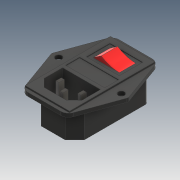
# Autodesk Inventor part: power-port
Saved by Autodesk Inventor 2017 (Build 210142000, 142)
## iProperties
Created: 2018-07-14
Part Number: power-port
Material: UHMW, Black
Document SubType Name: Modeling
Designer: Luiz Gustavo
Density: 0.94 g/cm^3
Appearance: Smooth - Black
Author: Luiz Gustavo
Autodesk Inventor part; units mm, degrees
ref_plane "YZ Plane" through (0, 0, 0) normal (1, 0, 0) x (0, 1, 0)
ref_plane "XZ Plane" through (0, 0, 0) normal (0, 1, 0) x (-1, 0, 0)
ref_plane "XY Plane" through (0, 0, 0) normal (0, 0, 1) x (1, 0, 0)
sketch "Sketch3" plane through (0, 0, 0) normal (0, 0, 1) x (1, 0, 0)
  line L0 (-13.75, 23.5) -> (13.75, 23.5)
  line L1 (13.75, 23.5) -> (13.75, -23.5)
  line L2 (13.75, -23.5) -> (-13.75, -23.5)
  line L3 (-13.75, -23.5) -> (-13.75, 23.5)
  line L4 (-13.75, 23.5) -> (13.75, -23.5) construction
  line L5 (13.75, 23.5) -> (-13.75, -23.5) construction
  point P0 (0, 0)
  dimension "d17" = 27.5
  dimension "d18" = 47
  constraints: 12 end point, 2 midpoint, 2 parallel, 1 horizontal, 1 perpendicular
  measures "d17" distance of L1.end L2.end
  measures "d18" distance between parallel lines of L2 L0
extrude "Extrusion1" add sketch "Sketch3" against normal blind 20
sketch "Sketch2" plane through (0, 0, 0) normal (0, 0, 1) x (1, 0, 0)
  line L0 (-24.5, 0) -> (24.5, 0) construction
  line L1 (0, 29.1) -> (0, -29.1) construction
  line L2 (-14, 29.1) -> (14, 29.1)
  line L3 (-14, 29.1) -> (-24.5, 0)
  line L4 (14, 29.1) -> (24.5, 0)
  line L5 (-14, -29.1) -> (14, -29.1)
  line L6 (-24.5, 0) -> (-14, -29.1)
  line L7 (24.5, 0) -> (14, -29.1)
  circle A0 centre (20, 0) radius 2
  circle A1 centre (-20, 0) radius 2
  point P0 (0, 0)
  point P1 (0, 0)
  dimension "d12" = 49
  dimension "d13" = 58.2
  dimension "d14" = 28
  dimension "d15" = 4
  dimension "d16" = 40
  constraints: 16 end point, 4 midpoint, 3 horizontal, 2 centre point, 2 point on line, 1 coincident, 1 equal radius, 1 parallel, 1 vertical, 1 other
  measures "d12" distance of L0.start L0.end
  measures "d13" distance of L1.start L1.end
  measures "d14" distance of L2.start L2.end
  measures "d15" diameter of A0
  measures "d16" distance of A1.centre A0.centre
extrude "Extrusion2" add sketch "Sketch2" against normal blind 2.3
sketch "Sketch1" plane through (0, 0, 0) normal (0, 0, 1) x (1, 0, 0)
  line L0 (-14.15, 27.2) -> (14.15, 27.2)
  line L1 (14.15, 27.2) -> (14.15, -27.2)
  line L2 (14.15, -27.2) -> (-14.15, -27.2)
  line L3 (-14.15, -27.2) -> (-14.15, 27.2)
  line L4 (-14.15, 27.2) -> (14.15, -27.2) construction
  line L5 (14.15, 27.2) -> (-14.15, -27.2) construction
  line L6 (-10.5, 23.2) -> (10.5, 23.2)
  line L7 (10.5, 23.2) -> (10.5, 8.2)
  line L8 (10.5, 8.2) -> (-10.5, 8.2)
  line L9 (-10.5, 8.2) -> (-10.5, 23.2)
  line L10 (-10.5, 23.2) -> (10.5, 8.2) construction
  line L11 (10.5, 23.2) -> (-10.5, 8.2) construction
  line L12 (0, 15.7) -> (0, 0) construction
  line L13 (-12.1, -5.4) -> (12.1, -5.4)
  line L14 (12.1, -5.4) -> (12.1, -22.2)
  line L15 (12.1, -22.2) -> (-12.1, -22.2)
  line L16 (-12.1, -22.2) -> (-12.1, -5.4)
  line L17 (-12.1, -5.4) -> (12.1, -22.2) construction
  line L18 (12.1, -5.4) -> (-12.1, -22.2) construction
  line L19 (0, 0) -> (0, -13.8) construction
  line L20 (-8.3, 20.95) -> (8.3, 20.95)
  line L21 (8.3, 20.95) -> (8.3, 10.45)
  line L22 (8.3, 10.45) -> (-8.3, 10.45)
  line L23 (-8.3, 10.45) -> (-8.3, 20.95)
  line L24 (-8.3, 20.95) -> (8.3, 10.45) construction
  line L25 (8.3, 20.95) -> (-8.3, 10.45) construction
  line L26 (-12.5, 5.8689) -> (12.5, 5.8689)
  line L27 (12.5, 5.8689) -> (12.5, -3.1311)
  line L28 (12.5, -3.1311) -> (-12.5, -3.1311)
  line L29 (-12.5, -3.1311) -> (-12.5, 5.8689)
  line L30 (-12.5, 5.8689) -> (12.5, -3.1311) construction
  line L31 (12.5, 5.8689) -> (-12.5, -3.1311) construction
  point P0 (0, 1.3689)
  dimension "d0" = 28.3
  dimension "d1" = 54.4
  dimension "d2" = 21
  dimension "d3" = 15
  dimension "d4" = 4
  dimension "d5" = 24.2
  dimension "d6" = 16.8
  dimension "d7" = 5
  dimension "d8" = 16.6
  dimension "d9" = 10.5
  dimension "d10" = 25
  dimension "d11" = 9
  constraints: 64 end point, 10 midpoint, 10 parallel, 5 horizontal, 5 perpendicular, 2 vertical, 1 point on line
  measures "d0" distance of L1.end L2.end
  measures "d1" distance of L0.end L1.end
  measures "d2" distance of L7.end L8.end
  measures "d3" distance of L6.end L7.end
  measures "d4" distance between parallel lines of L6 L0
  measures "d5" distance of L14.end L15.end
  measures "d6" distance of L13.end L14.end
  measures "d7" distance between parallel lines of L2 L15
  measures "d8" distance of L21.end L22.end
  measures "d9" distance of L20.end L21.end
  measures "d10" distance of L27.end L28.end
  measures "d11" distance of L26.end L27.end
extrude "Extrusion3" add sketch "Sketch1" along normal blind 1 contours L0 L1 L2 L3
extrude "Extrusion4" add sketch "Sketch1" along normal blind 0.5 contours L6 L7 L8 L9 | L26 L27 L28 L29
extrude "Extrusion5" add sketch "Sketch1" along normal blind 4 contours L20 L21 L22 L23
sketch "Sketch4" plane through (-8.3, 20.95, 0.5) normal (0, 1, 0) x (1, 0, 0)
  line L0 (0, -3.5) -> (16.6, -3.5) projected
  line L1 (0, 0) -> (0, -3.5) projected
  line L2 (16.6, 0) -> (16.6, -3.5) projected
  line L3 (0, 0) -> (5, -3.5)
  arc A0 (16.6, 0) -> (5, -3.5) centre (16.6082, -21) ccw
  point P0 (8.3, 0.5)
  dimension "d29" = 5
  dimension "d30" = 21
  constraints: 2 end point, 2 point on circle, 1 centre point, 1 point on line
  measures "d29" distance of L3.end L0.start
  measures "d30" radius of A0
extrude "Extrusion6" cut sketch "Sketch4" against normal up to surface (10.5 mm away)
extrude "Extrusion7" cut sketch "Sketch1" against normal blind 19 contours L13 L14 L15 L16
sketch "Sketch5" plane through (0, 0, 0) normal (0, 0, 1) x (1, 0, 0)
  line L0 (-1, -14.8319) -> (1, -14.8319)
  line L1 (1, -14.8319) -> (1, -18.3319)
  line L2 (1, -18.3319) -> (-1, -18.3319)
  line L3 (-1, -18.3319) -> (-1, -14.8319)
  line L4 (-8, -10.3319) -> (-6, -10.3319)
  line L5 (-6, -10.3319) -> (-6, -13.8319)
  line L6 (-6, -13.8319) -> (-8, -13.8319)
  line L7 (-8, -13.8319) -> (-8, -10.3319)
  line L8 (6, -10.3319) -> (8, -10.3319)
  line L9 (8, -10.3319) -> (8, -13.8319)
  line L10 (8, -13.8319) -> (6, -13.8319)
  line L11 (6, -13.8319) -> (6, -10.3319)
  line L12 (-8, -12.0819) -> (8, -12.0819) construction
  line L13 (0, -14.8319) -> (0, -12.0819) construction
  point P0 (0, 0)
  dimension "d35" = 2
  dimension "d36" = 3.5
  dimension "d42" = 16
  dimension "d43" = 8
  constraints: 28 end point, 10 parallel, 4 horizontal, 4 midpoint, 3 perpendicular, 1 vertical
  measures "d35" distance of L1.end L2.end
  measures "d36" distance of L0.end L1.end
  measures "d42" distance of L12.start L12.end
  measures "d43" distance between parallel lines of L2 L4
extrude "Extrusion8" add sketch "Sketch5" against normal up to next
fillet "Fillet1" radius 2 4 edges at (13.75, 23.5, -11.15) (-13.75, 23.5, -11.15) (24.5, 0, -1.15) (-24.5, 0, -1.15)
fillet "Fillet2" radius 5 4 edges at (14, 29.1, -1.15) (-14, 29.1, -1.15) (14, -29.1, -1.15) (-14, -29.1, -1.15)
chamfer "Chamfer1" distance 5 angle 45 2 edges at (12.1, -22.2, -9) (-12.1, -22.2, -9)
chamfer "Chamfer2" distance 6 angle 45 2 edges at (-13.75, -23.5, -11.15) (13.75, -23.5, -11.15)
body "Solid1"
